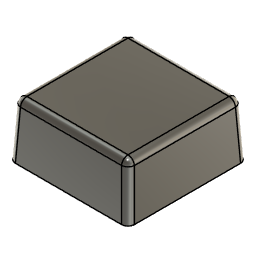
MX_Key_Template_Square v2 (Autodesk Fusion 360 design; units mm, degrees)
Autodesk Fusion 360 part; units mm, degrees
sketch "Sketch1" plane through (0, 0, 0) normal (0, 0, 1) x (1, 0, 0)
  line L0 (0, 0) -> (18.5, 0)
  line L1 (18.5, 0) -> (18.5, 18.5)
  line L2 (18.5, 18.5) -> (0, 18.5)
  line L3 (0, 18.5) -> (0, 0)
  dimension "d1" = 18.5
  dimension "d2" = 18.5
  constraint horizontal L0
  constraint vertical L1
  constraint horizontal L2
  constraint vertical L3
  constraint coincident L0.start L3.end
  measures "d1" distance of L0.start L0.end
  measures "d2" distance of L0.start L2.end
extrude "Extrude1" add sketch "Sketch1" along normal blind 8.5 makes body 1
draft "Draft1" angle -3 neutral plane through (0, 0, 0) pull (0, 0, -1) 1 faces at (18.5, 6.1667, 2.8333) on bodies 1
draft "Draft2" angle -3 neutral plane through (0, 0, 0) pull (0, 0, -1) 1 faces at (12.1848, 18.5, 2.8333) on bodies 1
draft "Draft3" angle -3 neutral plane through (0, 0, 0) pull (0, 0, -1) 1 faces at (0, 12.1848, 2.8333) on bodies 1
draft "Draft4" angle -3 neutral plane through (0, 0, 0) pull (0, 0, -1) 1 faces at (6.3152, 0, 2.8333) on bodies 1
fillet "Fillet1" radius 1 8 edges at (18.2773, 18.2773, 4.25) (0.2227, 18.2773, 4.25) (9.25, 18.0545, 8.5) (18.0545, 9.25, 8.5) (18.2773, 0.2227, 4.25) (9.25, 0.4455, 8.5) (0.4455, 9.25, 8.5) (0.2227, 0.2227, 4.25) on bodies 1
shell "Shell1" thickness 1 removed faces 1 at (12.3333, 6.4995, 0) on bodies 1
fillet "Fillet2" radius 0.5 4 edges at (1.1979, 1.1979, 3.75) (17.3021, 1.1979, 3.75) (17.3021, 17.3021, 3.75) (1.1979, 17.3021, 3.75) on bodies 1
sketch "Sketch2" plane through (0, 0, 7.5) normal (0, 0, -1) x (1, 0, 0)
  ellipse E0 centre (1.8951, -16.6049) end of major axis (1.5406, -16.9594) minor radius 0.5 (1.3944, -16.6063) -> (1.8937, -17.1056) ccw
  line L0 (1.8937, -17.1056) -> (16.6063, -17.1056)
  ellipse E1 centre (16.6049, -16.6049) end of major axis (16.9594, -16.9594) minor radius 0.5 (16.6063, -17.1056) -> (17.1056, -16.6063) ccw
  line L1 (17.1056, -16.6063) -> (17.1056, -1.8937)
  ellipse E2 centre (16.6049, -1.8951) end of major axis (16.9594, -1.5406) minor radius 0.5 (17.1056, -1.8937) -> (16.6063, -1.3944) ccw
  line L2 (16.6063, -1.3944) -> (1.8937, -1.3944)
  ellipse E3 centre (1.8951, -1.8951) end of major axis (1.5406, -1.5406) minor radius 0.5 (1.8937, -1.3944) -> (1.3944, -1.8937) ccw
  line L3 (1.3944, -1.8937) -> (1.3944, -16.6063)
  circle A0 centre (9.25, -9.25) radius 2.75
  dimension "d23" = 5.5
  measures "d23" diameter of A0
extrude "Extrude2" add sketch "Sketch2" along normal blind 5 contours A0 bodies 1
fillet "Fillet3" radius 2 1 edges at (6.6861, 8.2556, 7.5) on bodies 1
sketch "Sketch3" plane through (0, 0, 2.5) normal (0, 0, -1) x (1, 0, 0)
  circle A0 centre (9.25, -9.25) radius 2.75
  line L0 (9.885, -11.35) -> (8.615, -11.35)
  line L1 (8.615, -11.35) -> (8.615, -7.15)
  line L2 (8.615, -7.15) -> (9.885, -7.15)
  line L3 (9.885, -7.15) -> (9.885, -11.35)
  line L4 (11.35, -9.885) -> (7.15, -9.885)
  line L5 (7.15, -9.885) -> (7.15, -8.615)
  line L6 (7.15, -8.615) -> (11.35, -8.615)
  line L7 (11.35, -8.615) -> (11.35, -9.885)
  dimension "d29" = 2.1
  dimension "d30" = 2.1
  dimension "d31" = 0.635
  dimension "d32" = 0.635
  dimension "d33" = 0.635
  dimension "d34" = 0.635
  dimension "d35" = 2.1
  dimension "d36" = 2.1
  constraint horizontal L0
  constraint vertical L1
  constraint horizontal L2
  constraint vertical L3
  constraint horizontal L4
  constraint vertical L5
  constraint horizontal L6
  constraint vertical L7
  measures "d29" distance of A0.centre L0
  measures "d30" distance of A0.centre L2
  measures "d31" distance of A0.centre L3
  measures "d32" distance of A0.centre L1
  measures "d33" distance of A0.centre L4
  measures "d34" distance of A0.centre L6
  measures "d35" distance of A0.centre L7
  measures "d36" distance of A0.centre L5
extrude "Extrude3" cut sketch "Sketch3" against normal blind 5 contours L0 L1 L3 L4 | L1 L3 L4 L6 | L3 L4 L6 L7 | L1 L4 L5 L6 | L1 L2 L3 L6 bodies 1
sketch "Sketch4" plane through (0, 0, 2.5) normal (0, 0, -1) x (1, 0, 0)
  line L0 (9.885, -7.15) -> (9.885, -8.615)
  line L1 (9.885, -8.615) -> (11.35, -8.615)
  line L2 (11.35, -8.615) -> (11.35, -9.885)
  line L3 (11.35, -9.885) -> (9.885, -9.885)
  line L4 (9.885, -9.885) -> (9.885, -11.35)
  line L5 (9.885, -11.35) -> (8.615, -11.35)
  line L6 (8.615, -11.35) -> (8.615, -9.885)
  line L7 (8.615, -9.885) -> (7.15, -9.885)
  line L8 (7.15, -9.885) -> (7.15, -8.615)
  line L9 (7.15, -8.615) -> (8.615, -8.615)
  line L10 (8.615, -8.615) -> (8.615, -7.15)
  line L11 (8.615, -7.15) -> (9.885, -7.15)
  circle A0 centre (9.25, -9.25) radius 2.75
  line L12 (9.885, -11.35) -> (8.615, -11.35)
  line L13 (8.615, -11.35) -> (8.615, -13.35)
  line L14 (8.615, -13.35) -> (9.885, -13.35)
  line L15 (9.885, -13.35) -> (9.885, -11.35)
  line L16 (7.15, -9.885) -> (5.15, -9.885)
  line L17 (5.15, -9.885) -> (5.15, -8.615)
  line L18 (5.15, -8.615) -> (7.15, -8.615)
  line L19 (7.15, -8.615) -> (7.15, -9.885)
  line L20 (9.885, -7.15) -> (8.615, -7.15)
  line L21 (8.615, -7.15) -> (8.615, -5.15)
  line L22 (8.615, -5.15) -> (9.885, -5.15)
  line L23 (9.885, -5.15) -> (9.885, -7.15)
  line L24 (11.35, -8.615) -> (13.35, -8.615)
  line L25 (13.35, -8.615) -> (13.35, -9.885)
  line L26 (13.35, -9.885) -> (11.35, -9.885)
  line L27 (11.35, -9.885) -> (11.35, -8.615)
  dimension "d42" = 2
  dimension "d43" = 2
  dimension "d44" = 2
  dimension "d45" = 2
  constraint horizontal L12
  constraint vertical L13
  constraint horizontal L14
  constraint vertical L15
  constraint coincident L4.end L5.start
  constraint horizontal L16
  constraint vertical L17
  constraint horizontal L18
  constraint vertical L19
  constraint coincident L7.end L8.start
  constraint horizontal L20
  constraint vertical L21
  constraint horizontal L22
  constraint vertical L23
  constraint coincident L0.start L11.end
  constraint horizontal L24
  constraint vertical L25
  constraint horizontal L26
  constraint vertical L27
  constraint coincident L1.end L2.start
  measures "d42" distance of L4.end L14.end
  measures "d43" distance of L7.end L16.end
  measures "d44" distance of L1.end L24.end
  measures "d45" distance of L10.end L21.end
extrude "Extrude4" cut sketch "Sketch4" against normal blind 1.5 contours L11 A0 L20 L21 L23 | A0 L21 L22 L23 | L2 A0 L24 L26 L27 | A0 L24 L25 L26 | L8 A0 L16 L18 L19 | A0 L16 L17 L18 | L5 A0 L12 L13 L15 | A0 L13 L14 L15 bodies 1
fillet "Fillet4" radius 0.635 8 edges at (9.885, 11.6378, 4) (8.615, 11.6378, 4) (6.8622, 8.615, 4) (6.8622, 9.885, 4) (8.615, 6.8622, 4) (9.885, 6.8622, 4) (11.6378, 9.885, 4) (11.6378, 8.615, 4) on bodies 1
copy_body "Body->Comp1" bodies 1 removing the originals makes body 2 in component "Component"
component "Component" placed x (1, 0, 0) y (0, 1, 0) z (0, 0, 1) at (0, 0, 0)
equation "d1 = Width"
equation "d2 = Width"
equation "Height = 8.5 mm" comment "Button height"
equation "Width = 18.5 mm" comment "Button width"
equation "cornerRadius = 1 mm"
equation "sideAngle = 3 deg"
equation "wallThikcness = 1 mm"
equation "d8 = Height"
equation "d10 = -( sideAngle )"
equation "d12 = -( sideAngle )"
equation "d14 = -( sideAngle )"
equation "d16 = -( sideAngle )"
equation "d19 = cornerRadius"
equation "d20 = wallThikcness"
equation "d22 = cornerRadius / 2"
equation "knobHeight = 5 mm"
equation "d25 = knobHeight"
equation "d29 = crossLenght / 2"
equation "d30 = crossLenght / 2"
equation "d31 = crossWidth / 2"
equation "d32 = crossWidth / 2"
equation "d33 = crossWidth / 2"
equation "d34 = crossWidth / 2"
equation "d35 = crossLenght / 2"
equation "d36 = crossLenght / 2"
equation "d37 = -knobHeight"
equation "crossWidth = 1.27 mm"
equation "crossLenght = 4.2 mm"
equation "crossCut = 1.5 mm" comment "Cross cut depth"
equation "d46 = -crossCut"
equation "d49 = crossWidth / 2"
